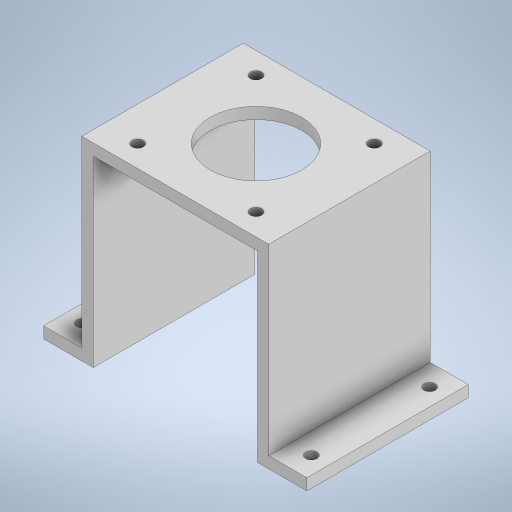
# Autodesk Inventor part: Motor_cage
Saved by Autodesk Inventor 2023 (Build 270158000, 158)
## iProperties
Created: 2022-12-10
Part Number: Motor_cage
Material: Generic
Document SubType Name: Modeling
Designer: Krzysztof
Density: 1 g/cm^3
Appearance: Default
Author: Krzysztof
## iProperties of the stored document Motor_cage_3DPrint.ipt
Created: 2022-12-19
Part Number: Motor_cage_3DPrint
Material: Generic
Document SubType Name: Modeling
Designer: Krzysztof
Density: 1 g/cm^3
Appearance: Default
Author: Krzysztof
Autodesk Inventor part; units mm, degrees
ref_plane "YZ Plane" through (0, 0, 0) normal (1, 0, 0) x (0, 1, 0)
ref_plane "XZ Plane" through (0, 0, 0) normal (0, 1, 0) x (-1, 0, 0)
ref_plane "XY Plane" through (0, 0, 0) normal (0, 0, 1) x (1, 0, 0)
sketch "Sketch1" plane through (0, 0, 0) normal (0, 1, 0) x (-1, 0, 0)
  line L0 (24.5, 21.15) -> (-24.5, 21.15)
  line L1 (-24.5, 21.15) -> (-24.5, -21.15)
  line L2 (-24.5, -21.15) -> (24.5, -21.15)
  line L3 (24.5, -21.15) -> (24.5, 21.15)
  line L4 (24.5, 21.15) -> (-24.5, -21.15) construction
  line L5 (-24.5, 21.15) -> (24.5, -21.15) construction
  circle A0 centre (0, 0) radius 12
  circle A1 centre (15.5, -15.5) radius 1.5
  line L6 (0, 0) -> (0, -30.8544) construction
  line L7 (0, 0) -> (-33.5596, 0) construction
  circle A2 centre (15.5, 15.5) radius 1.5
  circle A3 centre (-15.5, -15.5) radius 1.5
  circle A4 centre (-15.5, 15.5) radius 1.5
  dimension "d0" = 49
  dimension "d1" = 42.3
  dimension "d2" = 24
  dimension "d3" = 15.5
  dimension "d4" = 3
  dimension "d5" = 15.5
  dimension "d8" = 31
  dimension "d11" = 31
  constraints: 16 end point, 5 centre point, 3 horizontal, 2 midpoint, 2 parallel, 2 vertical, 1 coincident, 1 perpendicular, 6 other
  measures "d0" distance of L1.end L2.end
  measures "d1" distance of L0.end L1.end
  measures "d2" diameter of A0
  measures "d3" distance from line of L6 A1.centre
  measures "d4" diameter of A1
  measures "d5" distance from line of A1.centre L7
  measures "d8" distance of A1.centre A2.centre
  measures "d11" distance of A1.centre A3.centre
extrude "Extrusion1" add sketch "Sketch1" along normal blind 3
sketch "Sketch2" plane through (0, 0, 0) normal (0, -1, 0) x (1, 0, 0)
  line L0 (-24.5, 21.15) -> (24.5, 21.15) projected
  line L1 (24.5, -21.15) -> (-24.5, -21.15) projected
  line L2 (24.5, 21.15) -> (21.5, 21.15)
  line L3 (21.5, 21.15) -> (21.5, -21.15)
  line L4 (21.5, -21.15) -> (24.5, -21.15)
  line L5 (24.5, -21.15) -> (24.5, 21.15)
  point P0 (0, 0)
  dimension "d16" = 3
  constraints: 8 end point, 2 parallel, 1 horizontal, 1 perpendicular, 1 point on line
  measures "d16" distance between parallel lines of L5 L3
extrude "Extrusion2" add sketch "Sketch2" along normal blind 48
sketch "Sketch3" plane through (24.5, 3, 21.15) normal (1, 0, 0) x (0, 0, -1)
  line L0 (0, -51) -> (42.3, -51) projected
  line L1 (0, -51) -> (42.3, -51)
  line L2 (42.3, -51) -> (42.3, -48)
  line L3 (42.3, -48) -> (0, -48)
  line L4 (0, -48) -> (0, -51)
  point P0 (21.15, -3)
  dimension "d19" = 3
  constraints: 8 end point, 2 parallel, 1 horizontal, 1 perpendicular
  measures "d19" distance between parallel lines of L0 L3
extrude "Extrusion3" add sketch "Sketch3" along normal blind 10
sketch "Sketch4" plane through (24.5, -45, 21.15) normal (0, 1, 0) x (1, 0, 0)
  circle A0 centre (5.5, 36.65) radius 1.5
  circle A1 centre (-9, 36.65) radius 1.5 projected
  line L0 (-24.5, 21.15) -> (15.0504, 21.15) construction
  circle A2 centre (5.5, 5.65) radius 1.5
  dimension "d22" = 3
  dimension "d23" = 30
  constraints: 2 centre point, 2 end point, 1 horizontal, 1 horizontal alignment, 1 symmetric about line, 1 other
  measures "d22" diameter of A0
  measures "d23" horizontal distance of L0.start A0.centre
extrude "Extrusion4" cut sketch "Sketch4" against normal through all contours A0 | A2
mirror "Mirror1" about plane through (0, 0, 0) normal (1, 0, 0)
equation "\"d5\" = d3"
body "Solid1"
